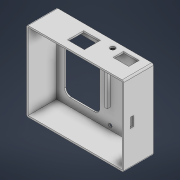
# Autodesk Inventor part: LightCasing
Saved by Autodesk Inventor 2021 (Build 250183000, 183)
## iProperties
Created: 2022-01-14
Part Number: LightCasing
Material: Generic
Document SubType Name: Sheet Metal
Designer: ivanl
Density: 1 g/cm^3
Appearance: Default
Sheet Metal Rule: Default
Author: ivanl
## iProperties of the stored document _3DPrint.ipt
Created: 2022-01-15
Part Number: _3DPrint
Material: Generic
Document SubType Name: Modeling
Designer: ivanl
Density: 1 g/cm^3
Appearance: Default
Author: ivanl
Autodesk Inventor part; units mm, degrees
ref_plane "YZ Plane" through (0, 0, 0) normal (1, 0, 0) x (0, 1, 0)
ref_plane "XZ Plane" through (0, 0, 0) normal (0, 1, 0) x (-1, 0, 0)
ref_plane "XY Plane" through (0, 0, 0) normal (0, 0, 1) x (1, 0, 0)
sketch "Sketch1" plane through (0, 0, 0) normal (0, 0, 1) x (1, 0, 0)
  line L0 (-60.5, -49.5) -> (60.5, -49.5)
  line L1 (60.5, -49.5) -> (60.5, 49.5)
  line L2 (60.5, 49.5) -> (-60.5, 49.5)
  line L3 (-60.5, 49.5) -> (-60.5, -49.5)
  line L4 (-60.5, -49.5) -> (60.5, 49.5) construction
  line L5 (60.5, -49.5) -> (-60.5, 49.5) construction
  point P0 (0, 0)
  dimension "d0" = 121
  dimension "d1" = 99
  constraints: 12 end point, 2 midpoint, 2 parallel, 1 horizontal, 1 perpendicular
  measures "d0" distance of L1.end L2.end
  measures "d1" distance of L0.end L1.end
extrude "Extrusion1" add sketch "Sketch1" along normal blind 37
sketch "Sketch3" plane through (0, 0, 37) normal (0, 0, 1) x (1, 0, 0)
  line L0 (-58.5, -47.5) -> (58.5, -47.5)
  line L1 (58.5, -47.5) -> (58.5, 47.5)
  line L2 (58.5, 47.5) -> (-58.5, 47.5)
  line L3 (-58.5, 47.5) -> (-58.5, -47.5)
  line L4 (-58.5, -47.5) -> (58.5, 47.5) construction
  line L5 (58.5, -47.5) -> (-58.5, 47.5) construction
  point P0 (0, 0)
  dimension "d8" = 117
  dimension "d9" = 95
  constraints: 12 end point, 2 midpoint, 2 parallel, 1 horizontal, 1 perpendicular
  measures "d8" distance of L1.end L2.end
  measures "d9" distance of L0.end L1.end
extrude "Extrusion3" cut sketch "Sketch3" against normal blind 35.3
sketch "Sketch4" plane through (0, 0, 1.7) normal (0, 0, 1) x (1, 0, 0)
  line L0 (5.5, -22.5) -> (8.5, -22.5)
  line L1 (8.5, -22.5) -> (8.5, 22.5)
  line L2 (8.5, 22.5) -> (5.5, 22.5)
  line L3 (5.5, 22.5) -> (5.5, -22.5)
  line L4 (5.5, -22.5) -> (8.5, 22.5) construction
  line L5 (8.5, -22.5) -> (5.5, 22.5) construction
  line L6 (-58.5, -47.5) -> (-58.5, 47.5) projected
  point P0 (0, 0)
  point P1 (7, 0)
  dimension "d12" = 3
  dimension "d13" = 65.5
  dimension "d14" = 45
  constraints: 12 end point, 2 midpoint, 2 parallel, 1 horizontal, 1 perpendicular
  measures "d12" distance of L1.end L2.end
  measures "d13" distance from line of L6 point (7, 0)
  measures "d14" distance of L0.end L1.end
extrude "Extrusion4" add sketch "Sketch4" along normal blind 4
sketch "Sketch5" plane through (-60.5, 49.5, 0) normal (0, -1, 0) x (1, 0, 0)
  circle A0 centre (79, 8.7) radius 3
  line L0 (119, 1.7) -> (2, 1.7) projected
  line L1 (69, 1.7) -> (69, 5.7) projected
  point P0 (60.5, 0)
  dimension "d17" = 6
  dimension "d18" = 7
  dimension "d19" = 10
  constraints: 1 centre point
  measures "d17" diameter of A0
  measures "d18" distance from line of L0 A0.centre
  measures "d19" distance from line of L1 A0.centre
extrude "Extrusion5" cut sketch "Sketch5" along normal blind 4
sketch "Sketch6" plane through (-60.5, 49.5, 0) normal (0, -1, 0) x (1, 0, 0)
  line L0 (89.25, 5.5) -> (108.75, 5.5)
  line L1 (108.75, 5.5) -> (108.75, 18.5)
  line L2 (108.75, 18.5) -> (89.25, 18.5)
  line L3 (89.25, 18.5) -> (89.25, 5.5)
  line L4 (89.25, 5.5) -> (108.75, 18.5) construction
  line L5 (108.75, 5.5) -> (89.25, 18.5) construction
  line L6 (0, 0) -> (121, 0) projected
  circle A0 centre (79, 8.7) radius 3 projected
  point P0 (60.5, 0)
  point P1 (99, 12)
  point P2 (79, 9)
  dimension "d23" = 19.5
  dimension "d24" = 13
  dimension "d25" = 12
  dimension "d26" = 20
  constraints: 12 end point, 2 midpoint, 2 parallel, 1 horizontal, 1 perpendicular
  measures "d23" distance of L1.end L2.end
  measures "d24" distance of L0.end L1.end
  measures "d25" distance from line of L6 point (99, 12)
  measures "d26" horizontal distance of point (79, 9) point (99, 12)
extrude "Extrusion6" cut sketch "Sketch6" along normal blind 4 contours L3 L2 L1 L0
sketch "Sketch9" plane through (60.5, -49.5, 0) normal (1, 0, 0) x (0, 0, -1)
  line L0 (-25, 43.5) -> (-29, 43.5)
  line L1 (-29, 43.5) -> (-29, 55.5)
  line L2 (-29, 55.5) -> (-25, 55.5)
  line L3 (-25, 55.5) -> (-25, 43.5)
  line L4 (-25, 43.5) -> (-29, 55.5) construction
  line L5 (-29, 43.5) -> (-25, 55.5) construction
  line L6 (-37, 0) -> (-37, 99) projected
  point P0 (0, 49.5)
  point P1 (-27, 49.5)
  point P2 (-27, 49.5)
  point P3 (-37, 49.5)
  dimension "d37" = 12
  dimension "d38" = 4
  dimension "d39" = 10
  constraints: 12 end point, 4 midpoint, 2 parallel, 1 horizontal, 1 horizontal alignment, 1 perpendicular
  measures "d37" distance of L0.end L1.end
  measures "d38" distance of L1.end L2.end
  measures "d39" distance from line of L6 point (-27, 49.5)
extrude "Extrusion8" cut sketch "Sketch9" against normal blind 10
fillet "Fillet2" radius 2 4 edges at (-60.5, -49.5, 18.5) (60.5, -49.5, 18.5) (60.5, 49.5, 18.5) (-60.5, 49.5, 18.5)
sketch "Sketch10" plane through (0, 0, 1.7) normal (0, 0, 1) x (1, 0, 0)
  line L0 (-48.5, 37.5) -> (-4.5, 37.5)
  line L1 (-4.5, 37.5) -> (-4.5, -37.5)
  line L2 (-4.5, -37.5) -> (-48.5, -37.5)
  line L3 (-48.5, -37.5) -> (-48.5, 37.5)
  line L4 (-48.5, 37.5) -> (-4.5, -37.5) construction
  line L5 (-4.5, 37.5) -> (-48.5, -37.5) construction
  line L6 (5.5, 22.5) -> (5.5, -22.5) projected
  line L7 (-58.5, -47.5) -> (-58.5, 47.5) projected
  line L8 (58.5, -47.5) -> (-58.5, -47.5) projected
  line L9 (-58.5, 47.5) -> (58.5, 47.5) projected
  point P0 (0, 0)
  point P1 (-26.5, 0)
  dimension "d43" = 10
  dimension "d44" = 10
  dimension "d45" = 10
  dimension "d46" = 10
  constraints: 12 end point, 2 midpoint, 2 parallel, 1 horizontal, 1 perpendicular
  measures "d43" distance between parallel lines of L6 L1
  measures "d44" distance between parallel lines of L7 L3
  measures "d45" distance between parallel lines of L8 L2
  measures "d46" distance between parallel lines of L9 L0
extrude "Extrusion9" cut sketch "Sketch10" against normal blind 10
sketch "Sketch12" plane through (-58.5, 49.5, 0) normal (0, 1, 0) x (1, 0, 0)
  line L0 (61, -28) -> (40, -28)
  line L1 (40, -28) -> (40, -8)
  line L2 (40, -8) -> (61, -8)
  line L3 (61, -8) -> (61, -28)
  line L4 (61, -28) -> (40, -8) construction
  line L5 (40, -28) -> (61, -8) construction
  line L6 (117, 0) -> (0, 0) projected
  point P0 (58.5, 0)
  point P1 (50.5, -18)
  point P2 (0, -37)
  dimension "d49" = 20
  dimension "d50" = 21
  dimension "d51" = 40
  dimension "d52" = 8
  constraints: 12 end point, 2 midpoint, 2 parallel, 1 horizontal, 1 perpendicular
  measures "d49" distance of L0.end L1.end
  measures "d50" distance of L0.start L0.end
  measures "d51" distance from line of point (0, -37) L1
  measures "d52" distance between parallel lines of L6 L2
extrude "Extrusion10" cut sketch "Sketch12" against normal blind 10
fillet "Fillet3" radius 7 4 edges at (-4.5, 37.5, 0.85) (-48.5, 37.5, 0.85) (-48.5, -37.5, 0.85) (-4.5, -37.5, 0.85)
sketch "Sketch13" plane through (0, 0, 1.7) normal (0, 0, 1) x (1, 0, 0)
  line L0 (58.5, 47.5) -> (58.5, -47.5) projected
  line L1 (-58.5, 47.5) -> (58.5, 47.5) projected
  line L2 (58.5, -47.5) -> (-58.5, -47.5) projected
  line L3 (-58.5, -47.5) -> (-58.5, 47.5) projected
  point P0 (0, 0)
  point P1 (8.5, -42.5)
  point P2 (8.5, 42.5)
  point P3 (8.5, 22.5)
  point P4 (8.5, -22.5)
  dimension "d57" = 5
  dimension "d58" = 5
  constraints: 2 vertical alignment
  measures "d57" distance from line of L1 point (8.5, 42.5)
  measures "d58" distance from line of L2 point (8.5, -42.5)
hole "Hole1" at (8.5, -42.5, 1.7) at (8.5, 42.5, 1.7) direction (0, 0, -1) diameter 4.496 end through all clearance for "Flat Head Machine Screw (82)" size "#8" standard "Ansi Unified Screw Threads"
equation "\"d65\" = Thickness"
equation "\"BendRadius\" = Thickness"
equation "\"BendReliefWidth\" = Thickness"
equation "\"BendReliefDepth\" = 0.5 * Thickness"
equation "\"CornerReliefSize\" = 4 * Thickness"
equation "\"MinimumRemnant\" = 2 * Thickness"
equation "\"TransitionRadius\" = BendRadius"
equation "\"JacobiRadiusSize\" = Thickness"
equation "\"GapSize\" = Thickness"
equation "\"Thickness\" = 0.5"
body "Solid1"
